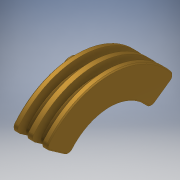
# Autodesk Inventor part: +XPanel_AntennaPost
Saved by Autodesk Inventor 2018 (Build 220112000, 112)
## iProperties
Created: 2018-10-28
Part Number: +XPanel_AntennaPost
Material: Brass, Soft Yellow
Document SubType Name: Modeling
Designer: Bradley
Density: 8.47 g/cm^3
Appearance: Brass - Satin
Mass: 0.744395 g
Surface Area: 1.99369 cm^2
Volume: 0.0878861 cm^3
Author: Bradley
Autodesk Inventor part; units mm, degrees
ref_plane "YZ Plane" through (0, 0, 0) normal (1, 0, 0) x (0, 1, 0)
ref_plane "XZ Plane" through (0, 0, 0) normal (0, 1, 0) x (-1, 0, 0)
ref_plane "XY Plane" through (0, 0, 0) normal (0, 0, 1) x (1, 0, 0)
sketch "Sketch3" plane through (0, 0, 0) normal (1, 0, 0) x (0, 1, 0)
  circle A0 centre (0, 0) radius 1
  dimension "d15" = 2
  constraints: 1 centre point, 1 coincident
  measures "d15" diameter of A0
extrude "Extrusion1" add sketch "Sketch3" along normal mid plane 0.6
sketch "Sketch4" plane through (0.3, 0, 0) normal (1, 0, 0) x (0, 0, -1)
  arc A0 (2.485, 5.7341) -> (2.485, -5.7341) centre (6.5, 0) ccw
  arc A1 (3.6321, 4.0958) -> (3.6321, -4.0958) centre (6.5, 0) ccw
  line L0 (-1.5, 0) -> (1.5, 0) construction
  line L1 (3.6321, -4.0958) -> (2.485, -5.7341)
  line L2 (2.485, 5.7341) -> (3.6321, 4.0958)
  arc A2 (1.9114, 6.5532) -> (1.9114, -6.5532) centre (6.5, 0) ccw
  line L3 (1.9114, 6.5532) -> (2.485, 5.7341)
  line L4 (2.485, -5.7341) -> (1.9114, -6.5532)
  point P0 (0, 0)
  point P1 (0, 0)
  dimension "d18" = 7
  dimension "d19" = 2
  dimension "d20" = 1
  dimension "d29" = 110
  constraints: 10 end point, 8 point on circle, 3 centre point, 2 collinear, 2 point on line, 1 coincident, 1 concentric, 1 horizontal, 1 midpoint
  measures "d18" radius of A0
  measures "d19" radial gap between concentric circles of A0 A1
  measures "d20" radial gap between concentric circles of A0 A2
  measures "d29" angle of L1 L2
extrude "Extrusion2" add sketch "Sketch4" along normal blind 0.5
extrude "Extrusion3" add sketch "Sketch4" along normal blind 3.5 contours L2 A1 L1 A0
pattern_linear "Rectangular Pattern1" count 3 spacing 1.5 along (1, 0, 0) of "Extrusion2"
fillet "Fillet1" radius 0.5 20 edges at (0.55, 6.5532, -1.9114) (1.3, 5.7341, -2.485) (2.05, 6.5532, -1.9114) (2.8, 5.7341, -2.485) (3.55, 6.5532, -1.9114) (0.55, 4.0958, -3.6321) (1.3, 4.0958, -3.6321) (2.05, 4.0958, -3.6321) (2.8, 4.0958, -3.6321) (3.55, 4.0958, -3.6321) (0.55, -4.0958, -3.6321) (1.3, -4.0958, -3.6321) (2.05, -4.0958, -3.6321) (2.8, -4.0958, -3.6321) (3.55, -4.0958, -3.6321) (3.55, -6.5532, -1.9114) (2.8, -5.7341, -2.485) (2.05, -6.5532, -1.9114) (1.3, -5.7341, -2.485) (0.55, -6.5532, -1.9114)
chamfer "Chamfer2" distance 0.1 angle 45 19 edges at (3.8, -6.3382, -1.8685) (3.8, 0, 1.5) (3.8, 6.3382, -1.8685) (3.8, 5.1104, -2.9217) (3.8, 5.932, -2.3464) (3.8, 4.1356, -3.4447) (3.8, 0, -1.5) (3.8, -4.1356, -3.4447) (3.8, -5.932, -2.3464) (3.8, -5.1104, -2.9217) (0.3, -5.3083, -2.7831) (0.3, -4.1356, -3.4447) (0.3, 0, -1.5) (0.3, -6.3382, -1.8685) (0.3, 0, 1.5) (0.3, 4.1356, -3.4447) (0.3, 5.3083, -2.7831) (0.3, 6.3382, -1.8685) (-0.3, -1, 0)
body "Solid2"
